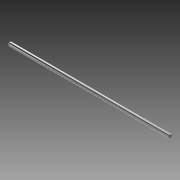
# Autodesk Inventor part: D-031
Saved by Autodesk Inventor 2015 (Build 190159000, 159)
## iProperties
Company: MARCHA TECHNOLOGY
Created: 2013-10-24
Part Number: D-031
Document SubType Name: Modeling
Designer: O.Martin
Density: 7.85 g/cm^3
Project: WITBOXprinter_K01
Material: Steel
Description: BARRA EJE Y
Stock Number: 28655
Mass: 140.017 g
Surface Area: 94.4125 cm^2
Volume: 17.8365 cm^3
Cost Center: 10
Appearance: Chrome - Polished Black
Author: O.Martin
Autodesk Inventor part; units mm, degrees
ref_plane "YZ Plane" through (0, 0, 0) normal (1, 0, 0) x (0, 1, 0)
ref_plane "XZ Plane" through (0, 0, 0) normal (0, 1, 0) x (-1, 0, 0)
ref_plane "XY Plane" through (0, 0, 0) normal (0, 0, 1) x (1, 0, 0)
sketch "Boceto1" plane through (0, 0, 0) normal (0, 0, 1) x (1, 0, 0)
  line L0 (-180, 4) -> (180, 4)
  line L1 (180, 4) -> (180, 0)
  line L2 (180, 0) -> (-180, 0)
  line L3 (-180, 0) -> (-180, 4)
  point P0 (0, 0)
  point P1 (0, 0)
  dimension "d0" = 8
  dimension "d1" = 360
  constraints: 8 end point, 2 parallel, 1 coincident, 1 horizontal, 1 midpoint, 1 perpendicular
  measures "d0" diameter of L0 L2
  measures "d1" distance of L1.end L2.end
revolve "Revolución1" add sketch "Boceto1" angle 360 about axis through (180, 0, 0) along (-1, 0, 0)
hole "Agujero1" at (-180, 0, 0) direction (1, 0, 0) diameter 3.242 depth 15 tip angle 118 thread size "M4x0.7" class "6H" standard "ISO Metric profile"
hole "Agujero2" at (180, 0, 0) direction (-1, 0, 0) diameter 3.242 depth 15 tip angle 118 thread size "M4x0.7" class "6H" standard "ISO Metric profile"
chamfer "Chaflán1" distance 0.5 angle 45 2 edges at (-180, -4, 0) (180, -4, 0)
body "Solid1"
